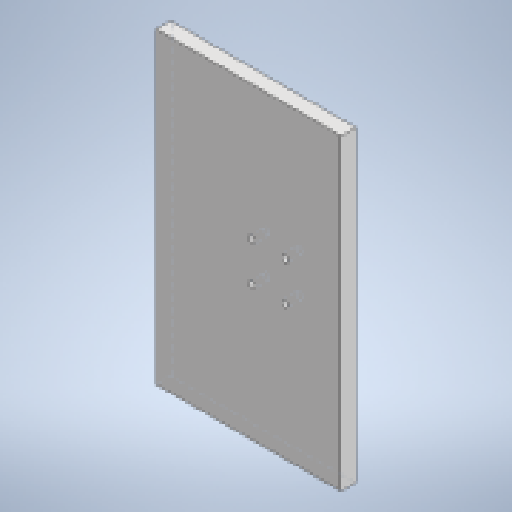
# Autodesk Inventor part: foot
Saved by Autodesk Inventor 2024 (Build 280153000, 153)
## iProperties
Created: 2024-09-17
Part Number: foot
Material: 일반
Document SubType Name: Modeling
Designer: Eungang
Density: 1 g/cm^3
Appearance: 기본값
Author: Eungang
Autodesk Inventor part; units mm, degrees
ref_plane "YZ Plane" through (0, 0, 0) normal (1, 0, 0) x (0, 1, 0)
ref_plane "XZ Plane" through (0, 0, 0) normal (0, 1, 0) x (-1, 0, 0)
ref_plane "XY Plane" through (0, 0, 0) normal (0, 0, 1) x (1, 0, 0)
sketch "스케치1" plane through (0, 0, 0) normal (0, 0, 1) x (1, 0, 0)
  circle A0 centre (15.05, -8.1625) radius 1.35 projected
  circle A1 centre (1.45, -8.1625) radius 1.35 projected
  circle A2 centre (15.05, 8.1625) radius 1.35 projected
  circle A3 centre (1.45, 8.1625) radius 1.35 projected
  line L0 (38.55, -64.25) -> (-38.55, -64.25) projected
  line L1 (38.55, 64.25) -> (38.55, -64.25) projected
  line L2 (-38.55, 64.25) -> (38.55, 64.25) projected
  line L3 (-38.55, -64.25) -> (-38.55, 64.25) projected
  point P0 (0, 0)
extrude "돌출1" add sketch "스케치1" against normal blind 6
